Support (Autodesk Fusion 360 design; units mm, degrees)
Autodesk Fusion 360 part; units mm, degrees
ref_plane "WorkPlane1" through (0, 0, 12.125) normal (0, 1, 0) x (0, 0, 1)
ref_plane "WorkPlane2" through (0, -124, 12.125) normal (0, 1, 0) x (0, 0, 1)
sketch "Sketch1" plane through (0, -124, 12.125) normal (0, 1, 0) x (0, 0, 1)
  circle A0 centre (332.231, -246.1613) radius 21
  line L0 (299.231, -270.1613) -> (299.231, -222.1613)
  line L1 (299.231, -270.1613) -> (334.0807, -267.0797)
  line L2 (299.231, -222.1613) -> (334.0807, -225.2429)
  line L3 (332.231, -246.1613) -> (299.231, -246.1613) construction
  point P0 (332.231, -246.1613)
  dimension "d3" = 42
  dimension "d5" = 48
  dimension "d6" = 33
  constraint coincident P0 A0.centre
  constraint coincident A0 L1.end
  constraint tangent A0 L1
  constraint coincident A0 L2.end
  constraint tangent A0 L2
  constraint vertical L0
  constraint midpoint L0 L3.end
  constraint perpendicular L0 L3
  measures "d3" diameter of A0
  measures "d5" distance of L0.end L0.start
  measures "d6" distance of L0 P0
extrude "Extrude1" add sketch "Sketch1" along normal blind 8 makes body 1
sketch "Sketch2" plane through (0, -116, 0) normal (0, 1, 0) x (-1, 0, 0)
  line L0 (270.1613, 311.356) -> (267.0797, 346.2057)
  arc A0 (267.0797, 346.2057) -> (225.2429, 346.2057) centre (246.1613, 344.356) ccw
  line L1 (225.2429, 346.2057) -> (222.1613, 311.356)
  line L2 (222.1613, 311.356) -> (270.1613, 311.356)
  line L3 (246.1613, 311.356) -> (246.1613, 365.356) construction
  circle A1 centre (246.1613, 351.356) radius 11.05
  circle A2 centre (246.1613, 351.356) radius 7
  line L4 (223.0456, 321.356) -> (269.277, 321.356) construction
  line L5 (232.1613, 321.356) -> (240.1613, 321.356)
  line L6 (240.1613, 321.356) -> (240.1613, 326.356)
  line L7 (240.1613, 326.356) -> (232.1613, 326.356)
  line L8 (232.1613, 326.356) -> (232.1613, 321.356)
  line L9 (260.1613, 326.356) -> (260.1613, 321.356)
  line L10 (260.1613, 321.356) -> (252.1613, 321.356)
  line L11 (252.1613, 326.356) -> (260.1613, 326.356)
  line L12 (252.1613, 321.356) -> (252.1613, 326.356)
  dimension "d10" = 22.1
  dimension "d11" = 40
  dimension "d14" = 14
  dimension "d23" = 10
  dimension "d24" = 8
  dimension "d25" = 5
  dimension "d27" = 6
  constraint midpoint L2 L3.start
  constraint midpoint A0 L3.end
  constraint coincident L3 A1.centre
  constraint concentric A1 A2
  constraint coincident L1 L4.start
  constraint coincident L0 L4.end
  constraint horizontal L4
  constraint horizontal L5
  constraint vertical L6
  constraint horizontal L7
  constraint vertical L8
  constraint coincident L4 L5.start
  constraint symmetric L3 L5.start L9.end
  constraint symmetric L3 L5.end L10.end
  constraint symmetric L3 L6.end L11.start
  constraint symmetric L3 L7.end L9.start
  measures "d10" diameter of A1
  measures "d11" distance of L3.start A1.centre
  measures "d14" diameter of A2
  measures "d23" vertical distance of L0.start L4.end
  measures "d24" distance of L6.end L7.end
  measures "d25" distance of L5.start L7.end
  measures "d27" horizontal distance of L3.start L5.end
extrude "Extrude2" cut sketch "Sketch2" against normal blind 7 contours A1 | L5 L6 L7 L8 | L9 L10 L11 L12 bodies 1
extrude "Extrude3" cut 1 faces at (-248.9102, -116, 349.7689) along direction (0, -1, 0) through all on bodies 1 bodies 1
sketch "Sketch3" plane through (0, 0, 311.356) normal (0, 0, -1) x (1, 0, 0)
  line L0 (-222.1613, 124) -> (-270.1613, 124)
  line L1 (-270.1613, 124) -> (-270.1613, 116)
  line L2 (-270.1613, 116) -> (-222.1613, 116)
  line L3 (-222.1613, 116) -> (-222.1613, 124)
  line L4 (-270.1613, 120) -> (-222.1613, 120) construction
  circle A0 centre (-256.1613, 120) radius 2.1
  circle A1 centre (-236.1613, 120) radius 2.1
  line L5 (-246.1613, 120) -> (-246.1613, 124) construction
  dimension "d16" = 4.2
  dimension "d17" = 4.2
  dimension "d19" = 10
  dimension "d20" = 10
  constraint midpoint L1 L4.start
  constraint midpoint L3 L4.end
  constraint coincident L4 A0.centre
  constraint coincident L4 A1.centre
  constraint midpoint L4 L5.start
  constraint midpoint L0 L5.end
  measures "d16" diameter of A0
  measures "d17" diameter of A1
  measures "d19" distance of A0.centre L5.start
  measures "d20" distance of A1.centre L5.start
extrude "Extrude4" cut sketch "Sketch3" against normal blind 15 contours A0 | A1 bodies 1
sketch "Sketch4" plane through (0, 0, 311.356) normal (0, 0, -1) x (1, 0, 0)
  circle A0 centre (-236.1613, 120) radius 2.1
  circle A1 centre (-256.1613, 120) radius 2.1
  line L0 (-222.1613, 124) -> (-270.1613, 124)
  line L1 (-270.1613, 124) -> (-270.1613, 116)
  line L2 (-270.1613, 116) -> (-222.1613, 116)
  line L3 (-222.1613, 116) -> (-222.1613, 124)
  line L4 (-270.1613, 124) -> (-270.1613, 97.5)
  line L5 (-270.1613, 124) -> (-222.1613, 124)
  line L6 (-222.1613, 124) -> (-222.1613, 97.5)
  line L7 (-270.1613, 97.5) -> (-222.1613, 97.5)
  line L8 (-270.1613, 116) -> (-222.1613, 97.5) construction
  line L9 (-246.1613, 106.75) -> (-270.1613, 106.75) construction
  line L10 (-246.1613, 106.75) -> (-222.1613, 106.75) construction
  circle A2 centre (-258.1613, 106.75) radius 2.1
  circle A3 centre (-234.1613, 106.75) radius 2.1
  dimension "d28" = 26.5
  dimension "d39" = 4.2
  dimension "d40" = 4.2
  constraint coincident L0.end L1.start
  constraint perpendicular L2 L4
  constraint coincident L0.start L3.end
  constraint perpendicular L0 L6
  constraint perpendicular L4 L7
  constraint coincident L1.end L2.start
  constraint midpoint L8 L9.start
  constraint coincident L4 L9.end
  constraint perpendicular L4 L9
  constraint perpendicular L6 L10
  constraint coincident L6 L10.end
  constraint midpoint L9 A2.centre
  constraint coincident L10 A3.centre
  constraint midpoint L10 A3.centre
  measures "d28" distance of L0.start L6.end
  measures "d39" diameter of A2
  measures "d40" diameter of A3
extrude "Extrude5" add sketch "Sketch4" along normal blind 11 separate body makes body 2
sketch "Sketch7" plane through (0, 0, 311.356) normal (0, 0, 1) x (-1, 0, 0)
  circle A0 centre (256.1613, 120) radius 2.1
  circle A1 centre (258.1613, 106.75) radius 2.1
  circle A2 centre (234.1613, 106.75) radius 2.1
  circle A3 centre (236.1613, 120) radius 2.1
  line L0 (270.1613, 97.5) -> (270.1613, 124)
  line L1 (270.1613, 124) -> (222.1613, 124)
  line L2 (222.1613, 124) -> (222.1613, 97.5)
  line L3 (222.1613, 97.5) -> (270.1613, 97.5)
  circle A4 centre (258.1613, 106.75) radius 3.5
  circle A5 centre (234.1613, 106.75) radius 3.5
  dimension "d46" = 7
  dimension "d47" = 7
  constraint concentric A1 A4
  constraint concentric A2 A5
  measures "d46" diameter of A4
  measures "d47" diameter of A5
sketch "Sketch8" plane through (0, 0, 300.356) normal (0, 0, -1) x (1, 0, 0)
  circle A0 centre (-256.1613, 120) radius 2.1
  circle A1 centre (-258.1613, 106.75) radius 2.1
  circle A2 centre (-234.1613, 106.75) radius 2.1
  circle A3 centre (-236.1613, 120) radius 2.1
  line L0 (-270.1613, 124) -> (-270.1613, 97.5)
  line L1 (-270.1613, 97.5) -> (-222.1613, 97.5)
  line L2 (-222.1613, 97.5) -> (-222.1613, 124)
  line L3 (-222.1613, 124) -> (-270.1613, 124)
  circle A4 centre (-256.1613, 120) radius 3.5
  circle A5 centre (-236.1613, 120) radius 3.5
  dimension "d42" = 7
  dimension "d43" = 7
  constraint concentric A0 A4
  constraint concentric A3 A5
  measures "d42" diameter of A4
  measures "d43" diameter of A5
extrude "Extrude8" cut sketch "Sketch7" against normal blind 3 contours A4 | A5 bodies 2
extrude "Extrude7" cut sketch "Sketch8" against normal blind 3 contours A4 | A5 bodies 2
mirror "Mirror1" about plane through (-270.1613, -97.5, 311.356) normal (0, 1, 0) of bodies 1 makes body 3
mirror "Mirror2" about plane through (-270.1613, -97.5, 311.356) normal (0, 1, 0) of bodies 2 makes body 4
combine "Combine1" operation add target body 2 tool bodies 4
